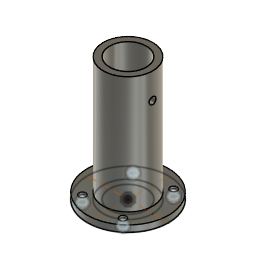
Tube Holder (Autodesk Fusion 360 design; units mm, degrees)
part number: 2026-03-26-20-08-00-795
Autodesk Fusion 360 part; units mm, degrees
sketch "Sketch1" plane through (0, 0, 0) normal (0, 0, 1) x (1, 0, 0)
  circle A0 centre (0, 0) radius 11.303
  circle A1 centre (0, 0) radius 25
  circle A2 centre (0, 0) radius 15.24
  circle A3 centre (-12.4939, 15.6174) radius 2.1209
  line L0 (0, 25) -> (0, -25) construction
  line L1 (-25, 0) -> (25, 0) construction
  line L2 (-25, 0) -> (25, 0) construction
  circle A4 centre (12.4939, 15.6174) radius 2.1209
  circle A5 centre (-12.4939, -15.6174) radius 2.1209
  circle A6 centre (12.4939, -15.6174) radius 2.1209
  dimension "d1" = 22.606
  dimension "d2" = 30.48
  dimension "d3" = 50
  dimension "d4" = 20
  dimension "d5" = 4.2418
  constraint coincident A0.centre A1.centre
  constraint concentric A0 A1
  constraint concentric A0 A2
  constraint coincident A1 L0.start
  constraint coincident A1 L0.end
  constraint vertical L0
  constraint coincident A1 L1.start
  constraint coincident A1 L1.end
  constraint perpendicular L0 L1
  constraint symmetric A3 L0 A4
  constraint symmetric A3 L2 A5
  constraint symmetric L2 A4 A6
  measures "d1" diameter of A0
  measures "d2" diameter of A2
  measures "d3" diameter of A1
  measures "d4" distance of A0.centre A3.centre
  measures "d5" diameter of A3
extrude "Extrude1" add sketch "Sketch1" along normal blind 4 contours A1
extrude "Extrude2" add sketch "Sketch1" along normal blind 76.2 contours A2
sketch "Sketch2" plane through (0, 0, 0) normal (1, 0, 0) x (0, 1, 0)
  circle A0 centre (0, 60.325) radius 2.1209
  dimension "d10" = 4.2418
  dimension "d11" = 60.325
  measures "d10" diameter of A0
  measures "d11" distance of A0.centre origin
extrude "Extrude3" cut sketch "Sketch2" along normal through all and the other way through all
